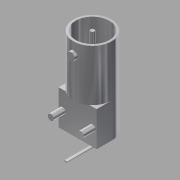
# Autodesk Inventor part: 0731000105
Saved by Autodesk Inventor 2013 (Build 170138000, 138)
## iProperties
Created: 2014-06-07
Part Number: 0731000105
Material: Generic
Document SubType Name: Modeling
Designer: Brad
Density: 1 g/cm^3
Author: Brad
Autodesk Inventor part; units mm, degrees
ref_plane "YZ Plane" through (0, 0, 0) normal (1, 0, 0) x (0, 1, 0)
sketch "Sketch1" plane through (0, 0, 0) normal (0, 0, 1) x (1, 0, 0)
  arc A0 (4.825, 0) -> (-4.825, 0) centre (0, 0) ccw
  line L0 (4.825, 0) -> (4.825, -3.775)
  line L1 (4.825, -3.775) -> (-4.825, -3.775)
  line L2 (-4.825, -3.775) -> (-4.825, 0)
  dimension "d0" = 9.65
  dimension "d2" = 3.775
  dimension "d3" = 9.65
  constraints: 6 end point, 2 point on circle, 2 tangent, 1 centre point, 1 coincident, 1 perpendicular, 1 vertical
  measures "d0" diameter of A0
  measures "d2" distance of L0.start L0.end
  measures "d3" distance of L0.end L1.end
extrude "Extrusion1" add sketch "Sketch1" along normal blind 8.8
sketch "Sketch2" plane through (0, 0, 8.8) normal (0, 0, 1) x (1, 0, 0)
  arc A0 (4.825, 0) -> (-4.825, 0) centre (0, 0) ccw projected
  circle A1 centre (0, 0) radius 4.825
  constraints: 1 centre point, 1 coincident, 1 concentric
extrude "Extrusion2" add sketch "Sketch2" along normal blind 13
ref_plane "Work Plane2" through (0, 0, 11.8) normal (0, 0, 1) x (1, 0, 0)
sketch "Sketch5" plane through (-4.825, -3.775, 0) normal (0, -1, 0) x (1, 0, 0)
  line L0 (1.82, 8.8) -> (7.83, 8.8) projected
  line L1 (0, 0) -> (0, 8.8) projected
  circle A0 centre (1.025, 4.2) radius 0.75
  circle A1 centre (8.625, 4.2) radius 0.75
  point P0 (4.825, 0)
  dimension "d15" = 1.5
  dimension "d17" = 1.5
  dimension "d18" = 4.6
  dimension "d19" = 4.6
  dimension "d20" = 7.6
  dimension "d21" = 1.025
  constraints: 2 centre point
  measures "d15" diameter of A0
  measures "d17" diameter of A1
  measures "d18" distance from line of A0.centre L0
  measures "d19" distance from line of L0 A1.centre
  measures "d20" distance of A1.centre A0.centre
  measures "d21" distance from line of L1 A0.centre
extrude "Extrusion5" add sketch "Sketch5" along normal blind 3
sketch "Sketch6" plane through (0, 0, 0) normal (0, 0, -1) x (-1, 0, 0)
  arc A0 (4.825, 0) -> (-4.825, 0) centre (0, 0) ccw projected
  circle A1 centre (0, 0) radius 1.75
  dimension "d24" = 3.5
  constraints: 1 centre point, 1 coincident
  measures "d24" diameter of A1
extrude "Extrusion6" add sketch "Sketch6" along normal blind 2
sketch "Sketch7" plane through (0, 0, -2) normal (0, 0, -1) x (-1, 0, 0)
  circle A0 centre (0, 0) radius 1.75 projected
  line L0 (-0.375, 0.15) -> (-0.375, -0.15)
  line L1 (-0.375, -0.15) -> (0.375, -0.15)
  line L2 (0.375, -0.15) -> (0.375, 0.15)
  line L3 (0.375, 0.15) -> (-0.375, 0.15)
  dimension "d28" = 0.3
  dimension "d30" = 0.75
  dimension "d31" = 0.375
  dimension "d32" = 0.15
  constraints: 8 end point, 2 parallel, 1 perpendicular, 1 vertical
  measures "d28" distance of L1.end L2.end
  measures "d30" distance of L0.end L1.end
  measures "d31" distance from line of A0.centre L2
  measures "d32" distance from line of A0.centre L3
extrude "Extrusion7" add sketch "Sketch7" along normal blind 1.75 contours L3 L2 L1 L0
sketch "Sketch8" plane through (-0.375, -0.15, -2) normal (0, -1, 0) x (1, 0, 0)
  line L0 (0, 0) -> (0, -1.75) projected
  line L1 (0.75, -1.75) -> (0, -1.75) projected
  line L2 (0.75, 0) -> (0.75, -1.75) projected
  line L3 (0, -1.75) -> (0, -1.45)
  line L4 (0, -1.45) -> (0.75, -1.45)
  line L5 (0.75, -1.45) -> (0.75, -1.75)
  line L6 (0, -1.75) -> (0.75, -1.75)
  point P0 (0.375, 2)
  dimension "d35" = 0.3
  dimension "d36" = 0.75
  constraints: 8 end point, 2 point on line, 1 parallel, 1 perpendicular
  measures "d35" distance of L0.end L3.end
  measures "d36" distance of L3.end L4.end
extrude "Extrusion8" add sketch "Sketch8" along normal blind 6.625
fillet "Fillet1" radius 0.2 1 edges at (1.75, 0, -2)
fillet "Fillet2" radius 0.1 9 edges at (-0.375, -3.3125, -3.75) (0.375, -3.3125, -3.75) (-0.375, -3.4625, -3.45) (0, 0.15, -3.75) (-0.375, 0.15, -2.875) (-0.375, -0.15, -2.725) (0.375, 0.15, -2.875) (0.375, -0.15, -2.725) (0.375, -3.4625, -3.45)
ref_plane "Work Plane1" through (0, 0, 21.8) normal (0, 1, 0) x (0, 0, 1)
sketch "Sketch9" plane through (0, 0, 21.8) normal (0, 1, 0) x (0, 0, 1)
  circle A0 centre (-3, 0) radius 1
  line L0 (0, -4.825) -> (0, 4.825) projected
  line L1 (0, 0) -> (-8.1755, 0)
  point P0 (-21.8, 0)
  dimension "d42" = 2
  dimension "d44" = 3
  dimension "d45" = 0
  constraints: 2 end point, 1 centre point, 1 midpoint, 1 perpendicular
  measures "d42" diameter of A0
  measures "d44" distance from line of L0 A0.centre
  measures "d45" distance from line of L1 A0.centre
extrude "Extrusion9" add sketch "Sketch9" along normal mid plane 11.02
sketch "Sketch3" plane through (0, 0, 21.8) normal (0, 0, 1) x (1, 0, 0)
  circle A0 centre (0, 0) radius 4.825 projected
  circle A1 centre (0, 0) radius 4.25
  dimension "d8" = 8.5
  constraints: 1 centre point, 1 coincident
  measures "d8" diameter of A1
extrude "Extrusion10" cut sketch "Sketch3" against normal blind 10 contours A1
sketch "Sketch4" plane through (0, 0, 11.8) normal (0, 0, 1) x (1, 0, 0)
  circle A0 centre (0, 0) radius 4.25 projected
  circle A1 centre (0, 0) radius 0.5
  dimension "d12" = 1
  constraints: 1 centre point, 1 coincident
  measures "d12" diameter of A1
extrude "Extrusion4" add sketch "Sketch4" along normal blind 10 contours A1
body "Solid1"
